Autodesk Inventor part; units mm, degrees
(part 3 of 4)
sketch "Sketch6" plane through (0, -25.4, 0) normal (0, -1, 0) x (1, 0, 0)
  line L0 (203.2, 0) -> (203.2, 304.8) projected
  line L1 (203.2, 304.8) -> (0, 304.8) projected
  line L2 (0, 304.8) -> (0, 0) projected
  line L3 (0, 0) -> (203.2, 0) projected
  line L4 (50.8, 88.9) -> (50.8, 215.9) construction
  line L5 (50.8, 215.9) -> (152.4, 215.9) construction
  line L6 (152.4, 215.9) -> (152.4, 88.9) construction
  line L7 (152.4, 88.9) -> (50.8, 88.9) construction
  spline S0 degree 2 poles (81.1955, 116.5983) (82.3959, 116.5983) (83.7001, 115.1312) (83.7001, 113.8937) knots 0 0 0 1 2 2 2
  spline S1 degree 2 poles (83.7001, 113.8937) (83.7001, 113.5973) (83.5964, 112.6117) (83.5223, 112.2783) knots 0 0 0 1 2 2 2
  line L8 (83.5223, 112.2783) -> (82.3515, 112.2783)
  line L9 (82.3515, 112.2783) -> (82.3515, 112.345)
  spline S2 degree 2 poles (82.3515, 112.345) (82.4404, 112.5969) (82.6479, 113.3453) (82.6479, 113.7307) knots 0 0 0 1 2 2 2
  spline S3 degree 2 poles (82.6479, 113.7307) (82.6479, 114.2938) (82.3885, 114.9681) (82.1514, 115.1237) knots 0 0 0 1 2 2 2
  spline S4 degree 2 poles (82.1514, 115.1237) (81.9069, 115.2942) (81.1955, 115.3831) (80.7287, 115.3831) knots 0 0 0 1 2 2 2
  line L10 (80.7287, 115.3831) -> (75.4009, 115.3831)
  line L11 (75.4009, 115.3831) -> (75.4009, 113.4491)
  line L12 (75.4009, 113.4491) -> (74.4301, 113.4491)
  line L13 (74.4301, 113.4491) -> (74.4301, 116.5983)
  line L14 (74.4301, 116.5983) -> (81.1955, 116.5983)
  spline S5 degree 2 poles (83.7668, 121.5853) (83.7668, 120.7776) (83.3444, 119.5772) (82.9221, 119.1548) knots 0 0 0 1 2 2 2
  spline S6 degree 2 poles (82.9221, 119.1548) (82.4478, 118.6732) (81.114, 118.2804) (80.1359, 118.2804) knots 0 0 0 1 2 2 2
  line L15 (80.1359, 118.2804) -> (74.4301, 118.2804)
  line L16 (74.4301, 118.2804) -> (74.4301, 119.4957)
  line L17 (74.4301, 119.4957) -> (80.1359, 119.4957)
  spline S7 degree 2 poles (80.1359, 119.4957) (80.7731, 119.4957) (81.6327, 119.6587) (81.981, 119.8884) knots 0 0 0 1 2 2 2
  spline S8 degree 2 poles (81.981, 119.8884) (82.3515, 120.1329) (82.7294, 120.9777) (82.7294, 121.5853) knots 0 0 0 1 2 2 2
  spline S9 degree 2 poles (82.7294, 121.5853) (82.7294, 122.1559) (82.3515, 123.0451) (81.981, 123.2896) knots 0 0 0 1 2 2 2
  spline S10 degree 2 poles (81.981, 123.2896) (81.6327, 123.5193) (80.7806, 123.6824) (80.1655, 123.6824) knots 0 0 0 1 2 2 2
  line L18 (80.1655, 123.6824) -> (74.4301, 123.6824)
  line L19 (74.4301, 123.6824) -> (74.4301, 124.8976)
  line L20 (74.4301, 124.8976) -> (80.1359, 124.8976)
  spline S11 degree 2 poles (80.1359, 124.8976) (81.0918, 124.8976) (82.4552, 124.5123) (82.9221, 124.0232) knots 0 0 0 1 2 2 2
  spline S12 degree 2 poles (82.9221, 124.0232) (83.3518, 123.586) (83.7668, 122.4301) (83.7668, 121.5853) knots 0 0 0 1 2 2 2
  spline S13 degree 2 poles (83.7372, 129.188) (83.7372, 128.1951) (83.3222, 126.802) (83.0258, 126.187) knots 0 0 0 1 2 2 2
  line L21 (83.0258, 126.187) -> (81.4993, 126.187)
  line L22 (81.4993, 126.187) -> (81.4993, 126.2759)
  spline S14 degree 2 poles (81.4993, 126.2759) (82.0625, 126.8761) (82.6849, 128.3951) (82.6849, 129.0991) knots 0 0 0 1 2 2 2
  spline S15 degree 2 poles (82.6849, 129.0991) (82.6849, 130.1069) (81.8476, 131.1369) (81.1585, 131.1369) knots 0 0 0 1 2 2 2
  spline S16 degree 2 poles (81.1585, 131.1369) (80.6101, 131.1369) (79.9284, 130.5959) (79.758, 130.0105) knots 0 0 0 1 2 2 2
  spline S17 degree 2 poles (79.758, 130.0105) (79.6394, 129.5882) (79.4764, 128.8842) (79.343, 128.3581) knots 0 0 0 1 2 2 2
  spline S18 degree 2 poles (79.343, 128.3581) (79.217, 127.8839) (78.8391, 127.1354) (78.5353, 126.8464) knots 0 0 0 1 2 2 2
  spline S19 degree 2 poles (78.5353, 126.8464) (78.2315, 126.5649) (77.4164, 126.2536) (76.8829, 126.2536) knots 0 0 0 1 2 2 2
  spline S20 degree 2 poles (76.8829, 126.2536) (75.7714, 126.2536) (74.2671, 127.9876) (74.2671, 129.3288) knots 0 0 0 1 2 2 2
  spline S21 degree 2 poles (74.2671, 129.3288) (74.2671, 130.0995) (74.5709, 131.4629) (74.8599, 132.0483) knots 0 0 0 1 2 2 2
  line L23 (74.8599, 132.0483) -> (76.3123, 132.0483)
  line L24 (76.3123, 132.0483) -> (76.3123, 131.9594)
  spline S22 degree 2 poles (76.3123, 131.9594) (75.9122, 131.5222) (75.3194, 130.1587) (75.3194, 129.4103) knots 0 0 0 1 2 2 2
  spline S23 degree 2 poles (75.3194, 129.4103) (75.3194, 128.5656) (76.1122, 127.5208) (76.7569, 127.5208) knots 0 0 0 1 2 2 2
  spline S24 degree 2 poles (76.7569, 127.5208) (77.3349, 127.5208) (78.024, 128.1358) (78.1796, 128.7138) knots 0 0 0 1 2 2 2
  spline S25 degree 2 poles (78.1796, 128.7138) (78.2834, 129.0991) (78.5501, 130.218) (78.6613, 130.5885) knots 0 0 0 1 2 2 2
  spline S26 degree 2 poles (78.6613, 130.5885) (78.9503, 131.5296) (80.1137, 132.404) (80.9658, 132.404) knots 0 0 0 1 2 2 2
  spline S27 degree 2 poles (80.9658, 132.404) (81.5067, 132.404) (82.5441, 131.9668) (82.9072, 131.5741) knots 0 0 0 1 2 2 2
  spline S28 degree 2 poles (82.9072, 131.5741) (83.3074, 131.1369) (83.7372, 130.0254) (83.7372, 129.188) knots 0 0 0 1 2 2 2
  line L25 (83.5741, 135.7756) -> (75.512, 135.7756)
  line L26 (75.512, 135.7756) -> (75.512, 132.7078)
  line L27 (75.512, 132.7078) -> (74.4301, 132.7078)
  line L28 (74.4301, 132.7078) -> (74.4301, 140.0586)
  line L29 (74.4301, 140.0586) -> (75.512, 140.0586)
  line L30 (75.512, 140.0586) -> (75.512, 136.9908)
  line L31 (75.512, 136.9908) -> (83.5741, 136.9908)
  line L32 (83.5741, 136.9908) -> (83.5741, 135.7756)
  line L33 (83.5741, 144.1711) -> (83.5741, 140.6291)
  line L34 (83.5741, 140.6291) -> (82.6405, 140.6291)
  line L35 (82.6405, 140.6291) -> (82.6405, 141.7925)
  line L36 (82.6405, 141.7925) -> (75.3638, 141.7925)
  line L37 (75.3638, 141.7925) -> (75.3638, 140.6291)
  line L38 (75.3638, 140.6291) -> (74.4301, 140.6291)
  line L39 (74.4301, 140.6291) -> (74.4301, 144.1711)
  line L40 (74.4301, 144.1711) -> (75.3638, 144.1711)
  line L41 (75.3638, 144.1711) -> (75.3638, 143.0078)
  line L42 (75.3638, 143.0078) -> (82.6405, 143.0078)
  line L43 (82.6405, 143.0078) -> (82.6405, 144.1711)
  line L44 (82.6405, 144.1711) -> (83.5741, 144.1711)
  line L45 (83.5741, 152.2185) -> (83.5741, 150.855)
  line L46 (83.5741, 150.855) -> (75.6899, 146.8091)
  line L47 (75.6899, 146.8091) -> (83.5741, 146.8091)
  line L48 (83.5741, 146.8091) -> (83.5741, 145.6754)
  line L49 (83.5741, 145.6754) -> (74.4301, 145.6754)
  line L50 (74.4301, 145.6754) -> (74.4301, 147.4019)
  line L51 (74.4301, 147.4019) -> (81.6698, 151.0847)
  line L52 (81.6698, 151.0847) -> (74.4301, 151.0847)
  line L53 (74.4301, 151.0847) -> (74.4301, 152.2185)
  line L54 (74.4301, 152.2185) -> (83.5741, 152.2185)
  line L55 (83.5741, 157.0128) -> (74.4301, 160.0953)
  line L56 (74.4301, 160.0953) -> (74.4301, 161.5922)
  line L57 (74.4301, 161.5922) -> (83.5741, 164.6747)
  line L58 (83.5741, 164.6747) -> (83.5741, 163.3928)
  line L59 (83.5741, 163.3928) -> (81.0177, 162.5629)
  line L60 (81.0177, 162.5629) -> (81.0177, 159.0727)
  line L61 (81.0177, 159.0727) -> (83.5741, 158.2428)
  line L62 (83.5741, 158.2428) -> (83.5741, 157.0128)
  line L63 (79.9803, 162.2294) -> (75.675, 160.8141)
  line L64 (75.675, 160.8141) -> (79.9803, 159.4062)
  line L65 (79.9803, 159.4062) -> (79.9803, 162.2294)
  line L66 (83.5741, 170.8399) -> (83.5741, 165.5417)
  line L67 (83.5741, 165.5417) -> (74.4301, 165.5417)
  line L68 (74.4301, 165.5417) -> (74.4301, 166.757)
  line L69 (74.4301, 166.757) -> (82.4923, 166.757)
  line L70 (82.4923, 166.757) -> (82.4923, 170.8399)
  line L71 (82.4923, 170.8399) -> (83.5741, 170.8399)
  line L72 (83.5741, 177.094) -> (83.5741, 171.7958)
  line L73 (83.5741, 171.7958) -> (74.4301, 171.7958)
  line L74 (74.4301, 171.7958) -> (74.4301, 173.011)
  line L75 (74.4301, 173.011) -> (82.4923, 173.011)
  line L76 (82.4923, 173.011) -> (82.4923, 177.094)
  line L77 (82.4923, 177.094) -> (83.5741, 177.094)
  line L78 (83.5741, 178.0499) -> (74.4301, 178.0499)
  line L79 (74.4301, 178.0499) -> (74.4301, 183.7704)
  line L80 (74.4301, 183.7704) -> (75.512, 183.7704)
  line L81 (75.512, 183.7704) -> (75.512, 179.2651)
  line L82 (75.512, 179.2651) -> (78.0166, 179.2651)
  line L83 (78.0166, 179.2651) -> (78.0166, 183.4666)
  line L84 (78.0166, 183.4666) -> (79.0985, 183.4666)
  line L85 (79.0985, 183.4666) -> (79.0985, 179.2651)
  line L86 (79.0985, 179.2651) -> (82.4923, 179.2651)
  line L87 (82.4923, 179.2651) -> (82.4923, 183.7704)
  line L88 (82.4923, 183.7704) -> (83.5741, 183.7704)
  line L89 (83.5741, 183.7704) -> (83.5741, 178.0499)
  line L90 (83.5741, 191.6473) -> (83.5741, 190.2839)
  line L91 (83.5741, 190.2839) -> (75.6899, 186.238)
  line L92 (75.6899, 186.238) -> (83.5741, 186.238)
  line L93 (83.5741, 186.238) -> (83.5741, 185.1042)
  line L94 (83.5741, 185.1042) -> (74.4301, 185.1042)
  line L95 (74.4301, 185.1042) -> (74.4301, 186.8308)
  line L96 (74.4301, 186.8308) -> (81.6698, 190.5136)
  line L97 (81.6698, 190.5136) -> (74.4301, 190.5136)
  line L98 (74.4301, 190.5136) -> (74.4301, 191.6473)
  line L99 (74.4301, 191.6473) -> (83.5741, 191.6473)
  line L100 (98.6295, 121.1222) -> (89.4855, 124.2048)
  line L101 (89.4855, 124.2048) -> (89.4855, 125.7016)
  line L102 (89.4855, 125.7016) -> (98.6295, 128.7842)
  line L103 (98.6295, 128.7842) -> (98.6295, 127.5022)
  line L104 (98.6295, 127.5022) -> (96.073, 126.6723)
  line L105 (96.073, 126.6723) -> (96.073, 123.1822)
  line L106 (96.073, 123.1822) -> (98.6295, 122.3523)
  line L107 (98.6295, 122.3523) -> (98.6295, 121.1222)
  line L108 (95.0356, 126.3389) -> (90.7304, 124.9235)
  line L109 (90.7304, 124.9235) -> (95.0356, 123.5156)
  line L110 (95.0356, 123.5156) -> (95.0356, 126.3389)
  line L111 (98.6295, 134.5714) -> (98.6295, 130.1106)
  line L112 (98.6295, 130.1106) -> (97.6958, 130.1106)
  line L113 (97.6958, 130.1106) -> (97.6958, 131.7704)
  line L114 (97.6958, 131.7704) -> (91.5677, 131.7704)
  line L115 (91.5677, 131.7704) -> (91.5677, 130.1106)
  line L116 (91.5677, 130.1106) -> (90.7304, 130.1106)
  spline S29 degree 2 poles (90.7304, 130.1106) (90.7304, 131.0516) (90.1969, 131.9409) (89.4559, 132.0001) knots 0 0 0 1 2 2 2
  line L117 (89.4559, 132.0001) -> (89.4559, 132.9486)
  line L118 (89.4559, 132.9486) -> (97.6958, 132.9486)
  line L119 (97.6958, 132.9486) -> (97.6958, 134.5714)
  line L120 (97.6958, 134.5714) -> (98.6295, 134.5714)
  line L121 (95.4876, 142.1371) -> (95.4876, 141.0478)
  line L122 (95.4876, 141.0478) -> (98.6295, 141.0478)
  line L123 (98.6295, 141.0478) -> (98.6295, 139.8696)
  line L124 (98.6295, 139.8696) -> (95.4876, 139.8696)
  line L125 (95.4876, 139.8696) -> (95.4876, 135.8311)
  line L126 (95.4876, 135.8311) -> (94.1983, 135.8311)
  line L127 (94.1983, 135.8311) -> (89.4855, 139.9215)
  line L128 (89.4855, 139.9215) -> (89.4855, 141.0478)
  line L129 (89.4855, 141.0478) -> (94.5021, 141.0478)
  line L130 (94.5021, 141.0478) -> (94.5021, 142.1371)
  line L131 (94.5021, 142.1371) -> (95.4876, 142.1371)
  line L132 (94.5021, 139.8696) -> (90.9305, 139.8696)
  line L133 (90.9305, 139.8696) -> (94.5021, 136.7944)
  line L134 (94.5021, 136.7944) -> (94.5021, 139.8696)
  spline S30 degree 2 poles (95.7248, 148.6579) (96.3843, 148.6579) (97.5106, 148.2356) (97.9255, 147.8502) knots 0 0 0 1 2 2 2
  spline S31 degree 2 poles (97.9255, 147.8502) (98.3405, 147.4649) (98.8222, 146.3163) (98.8222, 145.605) knots 0 0 0 1 2 2 2
  spline S32 degree 2 poles (98.8222, 145.605) (98.8222, 144.9529) (98.5332, 143.6784) (98.3035, 143.2115) knots 0 0 0 1 2 2 2
  line L135 (98.3035, 143.2115) -> (97.0067, 143.2115)
  line L136 (97.0067, 143.2115) -> (97.0067, 143.3005)
  spline S33 degree 2 poles (97.0067, 143.3005) (97.1104, 143.4412) (97.3772, 143.9674) (97.4958, 144.286) knots 0 0 0 1 2 2 2
  spline S34 degree 2 poles (97.4958, 144.286) (97.6217, 144.6491) (97.7625, 145.2493) (97.7625, 145.6272) knots 0 0 0 1 2 2 2
  spline S35 degree 2 poles (97.7625, 145.6272) (97.7625, 145.9977) (97.4958, 146.6943) (97.2068, 146.9462) knots 0 0 0 1 2 2 2
  spline S36 degree 2 poles (97.2068, 146.9462) (96.9326, 147.1759) (96.2064, 147.413) (95.7174, 147.413) knots 0 0 0 1 2 2 2
  spline S37 degree 2 poles (95.7174, 147.413) (95.2283, 147.413) (94.6058, 147.1463) (94.3984, 146.8943) knots 0 0 0 1 2 2 2
  spline S38 degree 2 poles (94.3984, 146.8943) (94.1687, 146.635) (93.976, 145.8643) (93.976, 145.3975) knots 0 0 0 1 2 2 2
  spline S39 degree 2 poles (93.976, 145.3975) (93.976, 144.8936) (94.1316, 143.8933) (94.1983, 143.5895) knots 0 0 0 1 2 2 2
  line L137 (94.1983, 143.5895) -> (89.4855, 143.5895)
  line L138 (89.4855, 143.5895) -> (89.4855, 148.6061)
  line L139 (89.4855, 148.6061) -> (90.56, 148.6061)
  line L140 (90.56, 148.6061) -> (90.56, 144.7676)
  line L141 (90.56, 144.7676) -> (92.9979, 144.7676)
  spline S40 degree 2 poles (92.9979, 144.7676) (92.9682, 144.9899) (92.946, 145.4197) (92.946, 145.5976) knots 0 0 0 1 2 2 2
  spline S41 degree 2 poles (92.946, 145.5976) (92.946, 146.3015) (93.1757, 147.2722) (93.5166, 147.7168) knots 0 0 0 1 2 2 2
  spline S42 degree 2 poles (93.5166, 147.7168) (93.8574, 148.1689) (94.8948, 148.6579) (95.7248, 148.6579) knots 0 0 0 1 2 2 2
  spline S43 degree 2 poles (95.6655, 155.7568) (96.3694, 155.7568) (97.5625, 155.2899) (97.9626, 154.8972) knots 0 0 0 1 2 2 2
  spline S44 degree 2 poles (97.9626, 154.8972) (98.385, 154.4896) (98.8222, 153.467) (98.8222, 152.852) knots 0 0 0 1 2 2 2
  spline S45 degree 2 poles (98.8222, 152.852) (98.8222, 152.237) (98.4072, 151.2218) (97.9922, 150.8365) knots 0 0 0 1 2 2 2
  spline S46 degree 2 poles (97.9922, 150.8365) (97.4958, 150.3622) (95.8285, 149.8287) (94.6133, 149.8287) knots 0 0 0 1 2 2 2
  spline S47 degree 2 poles (94.6133, 149.8287) (93.4202, 149.8287) (91.501, 150.3178) (90.7897, 150.8291) knots 0 0 0 1 2 2 2
  spline S48 degree 2 poles (90.7897, 150.8291) (90.0931, 151.3255) (89.3151, 152.8965) (89.3151, 153.9265) knots 0 0 0 1 2 2 2
  spline S49 degree 2 poles (89.3151, 153.9265) (89.3151, 154.2303) (89.3744, 154.7638) (89.441, 154.9639) knots 0 0 0 1 2 2 2
  line L142 (89.441, 154.9639) -> (90.6192, 154.9639)
  line L143 (90.6192, 154.9639) -> (90.6192, 154.912)
  spline S50 degree 2 poles (90.6192, 154.912) (90.5303, 154.7416) (90.3747, 154.1191) (90.3747, 153.7634) knots 0 0 0 1 2 2 2
  spline S51 degree 2 poles (90.3747, 153.7634) (90.3747, 152.6223) (91.916, 151.2218) (93.4276, 151.0884) knots 0 0 0 1 2 2 2
  spline S52 degree 2 poles (93.4276, 151.0884) (93.1238, 151.5256) (92.7904, 152.4445) (92.7904, 152.9928) knots 0 0 0 1 2 2 2
  spline S53 degree 2 poles (92.7904, 152.9928) (92.7904, 153.5263) (93.0053, 154.3266) (93.3313, 154.7638) knots 0 0 0 1 2 2 2
  spline S54 degree 2 poles (93.3313, 154.7638) (93.7092, 155.2677) (94.88, 155.7568) (95.6655, 155.7568) knots 0 0 0 1 2 2 2
  spline S55 degree 2 poles (95.7174, 154.5119) (95.1542, 154.5119) (94.391, 154.2155) (94.1242, 153.8894) knots 0 0 0 1 2 2 2
  spline S56 degree 2 poles (94.1242, 153.8894) (93.9315, 153.6449) (93.8056, 153.0373) (93.8056, 152.7186) knots 0 0 0 1 2 2 2
  spline S57 degree 2 poles (93.8056, 152.7186) (93.8056, 152.2888) (94.0649, 151.4812) (94.3094, 151.0884) knots 0 0 0 1 2 2 2
  spline S58 degree 2 poles (94.3094, 151.0884) (94.4428, 151.081) (94.6948, 151.0662) (94.8874, 151.0662) knots 0 0 0 1 2 2 2
  spline S59 degree 2 poles (94.8874, 151.0662) (95.8359, 151.0662) (96.9993, 151.4367) (97.3031, 151.7183) knots 0 0 0 1 2 2 2
  spline S60 degree 2 poles (97.3031, 151.7183) (97.5921, 151.9776) (97.8218, 152.5408) (97.8218, 152.8594) knots 0 0 0 1 2 2 2
  spline S61 degree 2 poles (97.8218, 152.8594) (97.8218, 153.6004) (96.7696, 154.5119) (95.7174, 154.5119) knots 0 0 0 1 2 2 2
  spline S62 degree 2 poles (95.6655, 162.6185) (96.3694, 162.6185) (97.5625, 162.1516) (97.9626, 161.7589) knots 0 0 0 1 2 2 2
  spline S63 degree 2 poles (97.9626, 161.7589) (98.385, 161.3513) (98.8222, 160.3288) (98.8222, 159.7137) knots 0 0 0 1 2 2 2
  spline S64 degree 2 poles (98.8222, 159.7137) (98.8222, 159.0987) (98.4072, 158.0835) (97.9922, 157.6982) knots 0 0 0 1 2 2 2
  spline S65 degree 2 poles (97.9922, 157.6982) (97.4958, 157.2239) (95.8285, 156.6904) (94.6133, 156.6904) knots 0 0 0 1 2 2 2
  spline S66 degree 2 poles (94.6133, 156.6904) (93.4202, 156.6904) (91.501, 157.1795) (90.7897, 157.6908) knots 0 0 0 1 2 2 2
  spline S67 degree 2 poles (90.7897, 157.6908) (90.0931, 158.1872) (89.3151, 159.7582) (89.3151, 160.7882) knots 0 0 0 1 2 2 2
  spline S68 degree 2 poles (89.3151, 160.7882) (89.3151, 161.092) (89.3744, 161.6255) (89.441, 161.8256) knots 0 0 0 1 2 2 2
  line L144 (89.441, 161.8256) -> (90.6192, 161.8256)
  line L145 (90.6192, 161.8256) -> (90.6192, 161.7737)
  spline S69 degree 2 poles (90.6192, 161.7737) (90.5303, 161.6033) (90.3747, 160.9808) (90.3747, 160.6252) knots 0 0 0 1 2 2 2
  spline S70 degree 2 poles (90.3747, 160.6252) (90.3747, 159.484) (91.916, 158.0835) (93.4276, 157.9501) knots 0 0 0 1 2 2 2
  spline S71 degree 2 poles (93.4276, 157.9501) (93.1238, 158.3873) (92.7904, 159.3062) (92.7904, 159.8545) knots 0 0 0 1 2 2 2
  spline S72 degree 2 poles (92.7904, 159.8545) (92.7904, 160.388) (93.0053, 161.1883) (93.3313, 161.6255) knots 0 0 0 1 2 2 2
  spline S73 degree 2 poles (93.3313, 161.6255) (93.7092, 162.1294) (94.88, 162.6185) (95.6655, 162.6185) knots 0 0 0 1 2 2 2
  spline S74 degree 2 poles (95.7174, 161.3736) (95.1542, 161.3736) (94.391, 161.0772) (94.1242, 160.7511) knots 0 0 0 1 2 2 2
  spline S75 degree 2 poles (94.1242, 160.7511) (93.9315, 160.5066) (93.8056, 159.899) (93.8056, 159.5803) knots 0 0 0 1 2 2 2
  spline S76 degree 2 poles (93.8056, 159.5803) (93.8056, 159.1506) (94.0649, 158.3429) (94.3094, 157.9501) knots 0 0 0 1 2 2 2
  spline S77 degree 2 poles (94.3094, 157.9501) (94.4428, 157.9427) (94.6948, 157.9279) (94.8874, 157.9279) knots 0 0 0 1 2 2 2
  spline S78 degree 2 poles (94.8874, 157.9279) (95.8359, 157.9279) (96.9993, 158.2984) (97.3031, 158.58) knots 0 0 0 1 2 2 2
  spline S79 degree 2 poles (97.3031, 158.58) (97.5921, 158.8393) (97.8218, 159.4025) (97.8218, 159.7211) knots 0 0 0 1 2 2 2
  spline S80 degree 2 poles (97.8218, 159.7211) (97.8218, 160.4621) (96.7696, 161.3736) (95.7174, 161.3736) knots 0 0 0 1 2 2 2
  spline S81 degree 2 poles (94.0575, 169.3912) (96.5176, 169.3912) (98.8222, 167.9611) (98.8222, 166.4717) knots 0 0 0 1 2 2 2
  spline S82 degree 2 poles (98.8222, 166.4717) (98.8222, 164.96) (96.4732, 163.5447) (94.0649, 163.5447) knots 0 0 0 1 2 2 2
  spline S83 degree 2 poles (94.0649, 163.5447) (91.59, 163.5447) (89.3002, 164.9749) (89.3002, 166.4717) knots 0 0 0 1 2 2 2
  spline S84 degree 2 poles (89.3002, 166.4717) (89.3002, 167.9759) (91.6715, 169.3912) (94.0575, 169.3912) knots 0 0 0 1 2 2 2
  spline S85 degree 2 poles (96.8437, 167.8203) (96.3917, 167.9982) (94.9986, 168.1464) (94.0575, 168.1464) knots 0 0 0 1 2 2 2
  spline S86 degree 2 poles (94.0575, 168.1464) (93.1164, 168.1464) (91.7307, 167.9982) (91.2639, 167.8129) knots 0 0 0 1 2 2 2
  spline S87 degree 2 poles (91.2639, 167.8129) (90.7971, 167.6276) (90.3154, 166.983) (90.3154, 166.4717) knots 0 0 0 1 2 2 2
  spline S88 degree 2 poles (90.3154, 166.4717) (90.3154, 165.9604) (90.7971, 165.3009) (91.2787, 165.1082) knots 0 0 0 1 2 2 2
  spline S89 degree 2 poles (91.2787, 165.1082) (91.7456, 164.923) (93.1683, 164.7896) (94.0649, 164.7896) knots 0 0 0 1 2 2 2
  spline S90 degree 2 poles (94.0649, 164.7896) (95.0282, 164.7896) (96.3176, 164.9082) (96.8214, 165.1008) knots 0 0 0 1 2 2 2
  spline S91 degree 2 poles (96.8214, 165.1008) (97.2957, 165.2787) (97.807, 165.9382) (97.807, 166.4717) knots 0 0 0 1 2 2 2
  spline S92 degree 2 poles (97.807, 166.4717) (97.807, 166.9756) (97.3253, 167.6351) (96.8437, 167.8203) knots 0 0 0 1 2 2 2
  line L146 (90.8564, 176.3048) -> (98.6295, 172.3478)
  line L147 (98.6295, 172.3478) -> (98.6295, 171.0437)
  line L148 (98.6295, 171.0437) -> (90.56, 175.2229)
  line L149 (90.56, 175.2229) -> (90.56, 170.5027)
  line L150 (90.56, 170.5027) -> (89.4855, 170.5027)
  line L151 (89.4855, 170.5027) -> (89.4855, 176.3048)
  line L152 (89.4855, 176.3048) -> (90.8564, 176.3048)
  line L153 (98.6295, 182.6034) -> (98.6295, 178.1425)
  line L154 (98.6295, 178.1425) -> (97.6958, 178.1425)
  line L155 (97.6958, 178.1425) -> (97.6958, 179.8024)
  line L156 (97.6958, 179.8024) -> (91.5677, 179.8024)
  line L157 (91.5677, 179.8024) -> (91.5677, 178.1425)
  line L158 (91.5677, 178.1425) -> (90.7304, 178.1425)
  spline S93 degree 2 poles (90.7304, 178.1425) (90.7304, 179.0836) (90.1969, 179.9728) (89.4559, 180.0321) knots 0 0 0 1 2 2 2
  line L159 (89.4559, 180.0321) -> (89.4559, 180.9806)
  line L160 (89.4559, 180.9806) -> (97.6958, 180.9806)
  line L161 (97.6958, 180.9806) -> (97.6958, 182.6034)
  line L162 (97.6958, 182.6034) -> (98.6295, 182.6034)
  spline S94 degree 2 poles (113.8775, 106.2724) (115.0483, 106.2724) (116.2784, 105.0127) (116.2784, 103.9086) knots 0 0 0 1 2 2 2
  spline S95 degree 2 poles (116.2784, 103.9086) (116.2784, 103.716) (116.2413, 103.2417) (116.2043, 103.012) knots 0 0 0 1 2 2 2
  line L163 (116.2043, 103.012) -> (115.1669, 103.012)
  line L164 (115.1669, 103.012) -> (115.1669, 103.0787)
  spline S96 degree 2 poles (115.1669, 103.0787) (115.1965, 103.2121) (115.2558, 103.5381) (115.2558, 103.6863) knots 0 0 0 1 2 2 2
  spline S97 degree 2 poles (115.2558, 103.6863) (115.2558, 104.1458) (115.0261, 104.746) (114.7815, 104.8868) knots 0 0 0 1 2 2 2
  spline S98 degree 2 poles (114.7815, 104.8868) (114.5592, 105.0276) (113.8849, 105.1165) (113.4033, 105.1165) knots 0 0 0 1 2 2 2
  line L165 (113.4033, 105.1165) -> (107.779, 105.1165)
  line L166 (107.779, 105.1165) -> (107.779, 103.879)
  line L167 (107.779, 103.879) -> (106.8232, 103.879)
  line L168 (106.8232, 103.879) -> (106.8232, 106.2724)
  line L169 (106.8232, 106.2724) -> (113.8775, 106.2724)
  line L170 (105.682, 106.2799) -> (105.682, 104.9683)
  line L171 (105.682, 104.9683) -> (104.4816, 104.9683)
  line L172 (104.4816, 104.9683) -> (104.4816, 106.2799)
  line L173 (104.4816, 106.2799) -> (105.682, 106.2799)
  spline S99 degree 2 poles (110.1429, 113.6973) (111.8249, 113.6973) (113.8775, 112.0671) (113.8775, 110.837) knots 0 0 0 1 2 2 2
  spline S100 degree 2 poles (113.8775, 110.837) (113.8775, 110.2813) (113.6033, 109.4884) (113.3662, 109.1031) knots 0 0 0 1 2 2 2
  line L174 (113.3662, 109.1031) -> (113.6849, 109.029)
  line L175 (113.6849, 109.029) -> (113.6849, 107.9471)
  line L176 (113.6849, 107.9471) -> (104.1333, 107.9471)
  line L177 (104.1333, 107.9471) -> (104.1333, 109.1031)
  line L178 (104.1333, 109.1031) -> (107.5419, 109.1031)
  spline S101 degree 2 poles (107.5419, 109.1031) (107.1492, 109.5403) (106.6305, 110.5555) (106.6305, 111.2001) knots 0 0 0 1 2 2 2
  spline S102 degree 2 poles (106.6305, 111.2001) (106.6305, 112.3635) (108.4904, 113.6973) (110.1429, 113.6973) knots 0 0 0 1 2 2 2
  spline S103 degree 2 poles (110.2318, 112.5043) (109.0017, 112.5043) (107.7272, 111.7559) (107.7272, 110.926) knots 0 0 0 1 2 2 2
  spline S104 degree 2 poles (107.7272, 110.926) (107.7272, 110.4591) (108.1718, 109.4958) (108.5126, 109.1031) knots 0 0 0 1 2 2 2
  line L179 (108.5126, 109.1031) -> (112.4474, 109.1031)
  spline S105 degree 2 poles (112.4474, 109.1031) (112.6623, 109.5403) (112.8401, 110.2146) (112.8401, 110.6147) knots 0 0 0 1 2 2 2
  spline S106 degree 2 poles (112.8401, 110.6147) (112.8401, 111.4965) (111.5878, 112.5043) (110.2318, 112.5043) knots 0 0 0 1 2 2 2
  spline S107 degree 2 poles (112.9587, 118.7213) (113.0624, 118.5805) (113.4329, 118.1063) (113.5441, 117.884) knots 0 0 0 1 2 2 2
  spline S108 degree 2 poles (113.5441, 117.884) (113.7071, 117.5802) (113.8775, 117.0096) (113.8775, 116.4909) knots 0 0 0 1 2 2 2
  spline S109 degree 2 poles (113.8775, 116.4909) (113.8775, 116.0685) (113.5589, 115.3053) (113.2699, 115.0163) knots 0 0 0 1 2 2 2
  spline S110 degree 2 poles (113.2699, 115.0163) (112.9883, 114.7421) (112.1584, 114.4087) (111.699, 114.4087) knots 0 0 0 1 2 2 2
  spline S111 degree 2 poles (111.699, 114.4087) (110.9876, 114.4087) (109.9798, 115.0089) (109.6908, 115.661) knots 0 0 0 1 2 2 2
  spline S112 degree 2 poles (109.6908, 115.661) (109.4241, 116.239) (109.224, 117.8099) (109.1721, 118.7213) knots 0 0 0 1 2 2 2
  line L180 (109.1721, 118.7213) -> (108.9498, 118.7213)
  spline S113 degree 2 poles (108.9498, 118.7213) (108.5497, 118.7213) (108.0532, 118.4768) (107.9124, 118.2545) knots 0 0 0 1 2 2 2
  spline S114 degree 2 poles (107.9124, 118.2545) (107.7716, 118.0322) (107.6827, 117.3949) (107.6827, 117.0541) knots 0 0 0 1 2 2 2
  spline S115 degree 2 poles (107.6827, 117.0541) (107.6827, 116.6539) (107.9198, 115.5721) (108.1495, 115.0311) knots 0 0 0 1 2 2 2
  line L181 (108.1495, 115.0311) -> (108.1495, 114.9644)
  line L182 (108.1495, 114.9644) -> (106.9714, 114.9644)
  spline S116 degree 2 poles (106.9714, 114.9644) (106.8824, 115.2831) (106.6601, 116.4761) (106.6601, 117.0615) knots 0 0 0 1 2 2 2
  spline S117 degree 2 poles (106.6601, 117.0615) (106.6601, 117.7728) (106.8824, 118.7436) (107.1714, 119.1289) knots 0 0 0 1 2 2 2
  spline S118 degree 2 poles (107.1714, 119.1289) (107.453, 119.5068) (108.3496, 119.8773) (108.9943, 119.8773) knots 0 0 0 1 2 2 2
  line L183 (108.9943, 119.8773) -> (113.6849, 119.8773)
  line L184 (113.6849, 119.8773) -> (113.6849, 118.7213)
  line L185 (113.6849, 118.7213) -> (112.9587, 118.7213)
  line L186 (111.9954, 118.7213) -> (110.091, 118.7213)
  spline S119 degree 2 poles (110.091, 118.7213) (110.128, 118.3064) (110.254, 117.0541) (110.3726, 116.6613) knots 0 0 0 1 2 2 2
  spline S120 degree 2 poles (110.3726, 116.6613) (110.5134, 116.2019) (111.0987, 115.6017) (111.6175, 115.6017) knots 0 0 0 1 2 2 2
  spline S121 degree 2 poles (111.6175, 115.6017) (112.2103, 115.6017) (112.8105, 116.2686) (112.8105, 116.9059) knots 0 0 0 1 2 2 2
  spline S122 degree 2 poles (112.8105, 116.9059) (112.8105, 117.4468) (112.3436, 118.336) (111.9954, 118.7213) knots 0 0 0 1 2 2 2
  line L187 (113.6849, 122.6783) -> (113.6849, 121.5223)
  line L188 (113.6849, 121.5223) -> (104.1333, 121.5223)
  line L189 (104.1333, 121.5223) -> (104.1333, 122.6783)
  line L190 (104.1333, 122.6783) -> (113.6849, 122.6783)
  line L191 (113.6849, 125.5534) -> (113.6849, 124.3974)
  line L192 (113.6849, 124.3974) -> (104.1333, 124.3974)
  line L193 (104.1333, 124.3974) -> (104.1333, 125.5534)
  line L194 (104.1333, 125.5534) -> (113.6849, 125.5534)
  spline S123 degree 2 poles (113.8405, 130.2291) (113.8405, 128.5841) (111.9954, 126.7761) (110.2911, 126.7761) knots 0 0 0 1 2 2 2
  spline S124 degree 2 poles (110.2911, 126.7761) (108.6164, 126.7761) (106.6305, 128.5322) (106.6305, 129.9476) knots 0 0 0 1 2 2 2
  spline S125 degree 2 poles (106.6305, 129.9476) (106.6305, 130.5848) (107.001, 131.5704) (107.3937, 131.9334) knots 0 0 0 1 2 2 2
  spline S126 degree 2 poles (107.3937, 131.9334) (107.7865, 132.3039) (108.9202, 132.6967) (109.7427, 132.6967) knots 0 0 0 1 2 2 2
  line L195 (109.7427, 132.6967) -> (110.3726, 132.6967)
  line L196 (110.3726, 132.6967) -> (110.3726, 127.9468)
  spline S127 degree 2 poles (110.3726, 127.9468) (111.5656, 127.9468) (112.8327, 129.1473) (112.8327, 130.2143) knots 0 0 0 1 2 2 2
  spline S128 degree 2 poles (112.8327, 130.2143) (112.8327, 130.5922) (112.6623, 131.3258) (112.5289, 131.6222) knots 0 0 0 1 2 2 2
  spline S129 degree 2 poles (112.5289, 131.6222) (112.3807, 131.9334) (112.1213, 132.3632) (112.0028, 132.504) knots 0 0 0 1 2 2 2
  line L197 (112.0028, 132.504) -> (112.0028, 132.5707)
  line L198 (112.0028, 132.5707) -> (113.2625, 132.5707)
  spline S130 degree 2 poles (113.2625, 132.5707) (113.344, 132.3706) (113.5811, 131.763) (113.6478, 131.5259) knots 0 0 0 1 2 2 2
  spline S131 degree 2 poles (113.6478, 131.5259) (113.7441, 131.1924) (113.8405, 130.6441) (113.8405, 130.2291) knots 0 0 0 1 2 2 2
  spline S132 degree 2 poles (109.4908, 131.5704) (109.0239, 131.5555) (108.3422, 131.3629) (108.1125, 131.1776) knots 0 0 0 1 2 2 2
  spline S133 degree 2 poles (108.1125, 131.1776) (107.8531, 130.9776) (107.579, 130.3477) (107.579, 129.8809) knots 0 0 0 1 2 2 2
  spline S134 degree 2 poles (107.579, 129.8809) (107.579, 129.4214) (107.8531, 128.7768) (108.1199, 128.51) knots 0 0 0 1 2 2 2
  spline S135 degree 2 poles (108.1199, 128.51) (108.3941, 128.2507) (109.0536, 127.9839) (109.4908, 127.9468) knots 0 0 0 1 2 2 2
  line L199 (109.4908, 127.9468) -> (109.4908, 131.5704)
  line L200 (113.6849, 139.2546) -> (113.6849, 138.0986)
  line L201 (113.6849, 138.0986) -> (109.7724, 138.0986)
  spline S136 degree 2 poles (109.7724, 138.0986) (109.2981, 138.0986) (108.483, 138.0097) (108.2385, 137.8763) knots 0 0 0 1 2 2 2
  spline S137 degree 2 poles (108.2385, 137.8763) (107.9791, 137.7355) (107.7272, 137.2316) (107.7272, 136.8018) knots 0 0 0 1 2 2 2
  spline S138 degree 2 poles (107.7272, 136.8018) (107.7272, 136.3721) (108.1866, 135.4606) (108.5571, 135.0234) knots 0 0 0 1 2 2 2
  line L202 (108.5571, 135.0234) -> (113.6849, 135.0234)
  line L203 (113.6849, 135.0234) -> (113.6849, 133.8675)
  line L204 (113.6849, 133.8675) -> (106.8232, 133.8675)
  line L205 (106.8232, 133.8675) -> (106.8232, 135.0234)
  line L206 (106.8232, 135.0234) -> (107.5864, 135.0234)
  spline S139 degree 2 poles (107.5864, 135.0234) (107.1196, 135.5421) (106.6305, 136.5425) (106.6305, 137.1057) knots 0 0 0 1 2 2 2
  spline S140 degree 2 poles (106.6305, 137.1057) (106.6305, 138.1134) (107.9643, 139.2546) (109.2314, 139.2546) knots 0 0 0 1 2 2 2
  line L207 (109.2314, 139.2546) -> (113.6849, 139.2546)
  spline S141 degree 2 poles (109.6093, 150.7179) (110.4615, 150.7179) (112.0546, 150.2511) (112.7141, 149.8139) knots 0 0 0 1 2 2 2
  line L208 (112.7141, 149.8139) -> (112.7141, 147.2352)
  line L209 (112.7141, 147.2352) -> (112.0028, 147.0796)
  spline S142 degree 2 poles (112.0028, 147.0796) (112.351, 146.6646) (112.766, 145.9755) (112.766, 145.3753) knots 0 0 0 1 2 2 2
  spline S143 degree 2 poles (112.766, 145.3753) (112.766, 144.4342) (111.2469, 143.2264) (109.8094, 143.2264) knots 0 0 0 1 2 2 2
  spline S144 degree 2 poles (109.8094, 143.2264) (108.3644, 143.2264) (106.7565, 144.7084) (106.7565, 145.6643) knots 0 0 0 1 2 2 2
  spline S145 degree 2 poles (106.7565, 145.6643) (106.7565, 146.1089) (106.9788, 146.7461) (107.164, 147.0722) knots 0 0 0 1 2 2 2
  line L210 (107.164, 147.0722) -> (106.8676, 147.0722)
  line L211 (106.8676, 147.0722) -> (106.8676, 148.0429)
  line L212 (106.8676, 148.0429) -> (112.0324, 148.0429)
  line L213 (112.0324, 148.0429) -> (112.0324, 149.436)
  spline S146 degree 2 poles (112.0324, 149.436) (111.5952, 149.6731) (110.2095, 149.8732) (109.6464, 149.8732) knots 0 0 0 1 2 2 2
  spline S147 degree 2 poles (109.6464, 149.8732) (107.6383, 149.8732) (105.1929, 147.828) (105.1929, 145.9088) knots 0 0 0 1 2 2 2
  spline S148 degree 2 poles (105.1929, 145.9088) (105.1929, 144.0933) (107.8383, 141.7295) (109.7279, 141.7295) knots 0 0 0 1 2 2 2
  spline S149 degree 2 poles (109.7279, 141.7295) (111.7508, 141.7295) (114.2628, 144.0266) (114.2628, 145.8792) knots 0 0 0 1 2 2 2
  spline S150 degree 2 poles (114.2628, 145.8792) (114.2628, 146.3756) (114.1295, 147.4797) (113.9813, 147.9688) knots 0 0 0 1 2 2 2
  line L214 (113.9813, 147.9688) -> (114.8482, 147.9688)
  spline S151 degree 2 poles (114.8482, 147.9688) (114.9742, 147.4501) (115.0705, 146.3905) (115.0705, 145.8717) knots 0 0 0 1 2 2 2
  spline S152 degree 2 poles (115.0705, 145.8717) (115.0705, 143.7006) (112.0843, 140.8477) (109.7131, 140.8477) knots 0 0 0 1 2 2 2
  spline S153 degree 2 poles (109.7131, 140.8477) (107.4604, 140.8477) (104.363, 143.7895) (104.363, 145.9014) knots 0 0 0 1 2 2 2
  spline S154 degree 2 poles (104.363, 145.9014) (104.363, 148.1615) (107.2752, 150.7179) (109.6093, 150.7179) knots 0 0 0 1 2 2 2
  line L215 (111.1803, 147.0574) -> (108.0013, 147.0574)
  spline S155 degree 2 poles (108.0013, 147.0574) (107.8235, 146.7165) (107.6679, 146.1385) (107.6679, 145.8199) knots 0 0 0 1 2 2 2
  spline S156 degree 2 poles (107.6679, 145.8199) (107.6679, 145.1233) (108.7053, 144.2786) (109.7946, 144.2786) knots 0 0 0 1 2 2 2
  spline S157 degree 2 poles (109.7946, 144.2786) (110.7727, 144.2786) (111.8175, 144.9159) (111.8175, 145.6198) knots 0 0 0 1 2 2 2
  spline S158 degree 2 poles (111.8175, 145.6198) (111.8175, 145.9903) (111.4618, 146.7239) (111.1803, 147.0574) knots 0 0 0 1 2 2 2
  line L216 (113.6849, 157.6463) -> (113.6849, 156.4903)
  line L217 (113.6849, 156.4903) -> (112.929, 156.4903)
  spline S159 degree 2 poles (112.929, 156.4903) (113.3959, 155.9568) (113.8775, 155.0009) (113.8775, 154.4081) knots 0 0 0 1 2 2 2
  spline S160 degree 2 poles (113.8775, 154.4081) (113.8775, 153.9635) (113.5811, 153.1706) (113.2625, 152.8817) knots 0 0 0 1 2 2 2
  spline S161 degree 2 poles (113.2625, 152.8817) (112.9439, 152.5853) (111.9731, 152.2592) (111.2766, 152.2592) knots 0 0 0 1 2 2 2
  line L218 (111.2766, 152.2592) -> (106.8232, 152.2592)
  line L219 (106.8232, 152.2592) -> (106.8232, 153.4152)
  line L220 (106.8232, 153.4152) -> (110.7357, 153.4152)
  spline S162 degree 2 poles (110.7357, 153.4152) (111.284, 153.4152) (112.0028, 153.4967) (112.2695, 153.6375) knots 0 0 0 1 2 2 2
  spline S163 degree 2 poles (112.2695, 153.6375) (112.5363, 153.7783) (112.7808, 154.2599) (112.7808, 154.7119) knots 0 0 0 1 2 2 2
  spline S164 degree 2 poles (112.7808, 154.7119) (112.7808, 155.1343) (112.2992, 156.0902) (111.9509, 156.4903) knots 0 0 0 1 2 2 2
  line L221 (111.9509, 156.4903) -> (106.8232, 156.4903)
  line L222 (106.8232, 156.4903) -> (106.8232, 157.6463)
  line L223 (106.8232, 157.6463) -> (113.6849, 157.6463)
  spline S165 degree 2 poles (113.8405, 162.0479) (113.8405, 161.3365) (113.4033, 160.1583) (112.9587, 159.7359) knots 0 0 0 1 2 2 2
  spline S166 degree 2 poles (112.9587, 159.7359) (112.5215, 159.3136) (111.1728, 158.8467) (110.2688, 158.8467) knots 0 0 0 1 2 2 2
  spline S167 degree 2 poles (110.2688, 158.8467) (109.3648, 158.8467) (108.0458, 159.3284) (107.6012, 159.7359) knots 0 0 0 1 2 2 2
  spline S168 degree 2 poles (107.6012, 159.7359) (107.1492, 160.1435) (106.6675, 161.3513) (106.6675, 162.0479) knots 0 0 0 1 2 2 2
  spline S169 degree 2 poles (106.6675, 162.0479) (106.6675, 162.611) (106.9862, 163.6633) (107.1937, 164.0708) knots 0 0 0 1 2 2 2
  line L224 (107.1937, 164.0708) -> (108.4904, 164.0708)
  line L225 (108.4904, 164.0708) -> (108.4904, 164.0041)
  spline S170 degree 2 poles (108.4904, 164.0041) (108.3867, 163.8782) (108.1199, 163.4928) (107.9791, 163.2187) knots 0 0 0 1 2 2 2
  spline S171 degree 2 poles (107.9791, 163.2187) (107.8606, 162.9741) (107.6753, 162.3221) (107.6753, 162.0257) knots 0 0 0 1 2 2 2
  spline S172 degree 2 poles (107.6753, 162.0257) (107.6753, 161.129) (109.0313, 160.0398) (110.2688, 160.0398) knots 0 0 0 1 2 2 2
  spline S173 degree 2 poles (110.2688, 160.0398) (111.4767, 160.0398) (112.8327, 161.092) (112.8327, 162.0257) knots 0 0 0 1 2 2 2
  spline S174 degree 2 poles (112.8327, 162.0257) (112.8327, 162.5888) (112.3659, 163.6114) (112.0028, 164.0041) knots 0 0 0 1 2 2 2
  line L226 (112.0028, 164.0041) -> (112.0028, 164.0708)
  line L227 (112.0028, 164.0708) -> (113.2995, 164.0708)
  spline S175 degree 2 poles (113.2995, 164.0708) (113.381, 163.9004) (113.6108, 163.3817) (113.6626, 163.1742) knots 0 0 0 1 2 2 2
  spline S176 degree 2 poles (113.6626, 163.1742) (113.7515, 162.8778) (113.8405, 162.411) (113.8405, 162.0479) knots 0 0 0 1 2 2 2
  spline S177 degree 2 poles (113.8479, 166.9756) (113.8479, 166.2864) (113.4774, 165.0934) (113.2699, 164.7007) knots 0 0 0 1 2 2 2
  line L228 (113.2699, 164.7007) -> (111.9731, 164.7007)
  line L229 (111.9731, 164.7007) -> (111.9731, 164.76)
  spline S178 degree 2 poles (111.9731, 164.76) (112.0917, 164.9082) (112.3733, 165.3083) (112.5289, 165.6418) knots 0 0 0 1 2 2 2
  spline S179 degree 2 poles (112.5289, 165.6418) (112.6697, 165.9307) (112.8772, 166.6421) (112.8772, 167.02) knots 0 0 0 1 2 2 2
  spline S180 degree 2 poles (112.8772, 167.02) (112.8772, 167.2942) (112.7512, 167.9241) (112.6474, 168.0723) knots 0 0 0 1 2 2 2
  spline S181 degree 2 poles (112.6474, 168.0723) (112.5067, 168.2871) (112.188, 168.4798) (111.862, 168.4798) knots 0 0 0 1 2 2 2
  spline S182 degree 2 poles (111.862, 168.4798) (111.4544, 168.4798) (111.0321, 168.0352) (110.8913, 167.4646) knots 0 0 0 1 2 2 2
  spline S183 degree 2 poles (110.8913, 167.4646) (110.8394, 167.2423) (110.6912, 166.531) (110.6097, 166.2272) knots 0 0 0 1 2 2 2
  spline S184 degree 2 poles (110.6097, 166.2272) (110.38, 165.4417) (109.4315, 164.7303) (108.7572, 164.7303) knots 0 0 0 1 2 2 2
  spline S185 degree 2 poles (108.7572, 164.7303) (107.8235, 164.7303) (106.6601, 166.1308) (106.6601, 167.2868) knots 0 0 0 1 2 2 2
  spline S186 degree 2 poles (106.6601, 167.2868) (106.6601, 167.8574) (106.9417, 169.0133) (107.1566, 169.4061) knots 0 0 0 1 2 2 2
  line L230 (107.1566, 169.4061) -> (108.3941, 169.4061)
  line L231 (108.3941, 169.4061) -> (108.3941, 169.3468)
  spline S187 degree 2 poles (108.3941, 169.3468) (108.0384, 168.9022) (107.6308, 167.8203) (107.6308, 167.2646) knots 0 0 0 1 2 2 2
  spline S188 degree 2 poles (107.6308, 167.2646) (107.6308, 166.694) (108.1125, 165.9085) (108.5942, 165.9085) knots 0 0 0 1 2 2 2
  spline S189 degree 2 poles (108.5942, 165.9085) (109.0313, 165.9085) (109.4537, 166.3754) (109.5871, 166.8941) knots 0 0 0 1 2 2 2
  spline S190 degree 2 poles (109.5871, 166.8941) (109.6538, 167.146) (109.7872, 167.7833) (109.8687, 168.1315) knots 0 0 0 1 2 2 2
  spline S191 degree 2 poles (109.8687, 168.1315) (110.0613, 168.8874) (110.9431, 169.658) (111.7064, 169.658) knots 0 0 0 1 2 2 2
  spline S192 degree 2 poles (111.7064, 169.658) (112.151, 169.658) (112.9364, 169.3097) (113.2254, 168.9689) knots 0 0 0 1 2 2 2
  spline S193 degree 2 poles (113.2254, 168.9689) (113.5292, 168.6058) (113.8479, 167.6795) (113.8479, 166.9756) knots 0 0 0 1 2 2 2
  line L232 (113.6849, 176.0084) -> (113.6849, 174.8524)
  line L233 (113.6849, 174.8524) -> (112.9883, 174.8524)
  spline S194 degree 2 poles (112.9883, 174.8524) (113.2106, 174.5857) (113.507, 174.193) (113.633, 173.9262) knots 0 0 0 1 2 2 2
  spline S195 degree 2 poles (113.633, 173.9262) (113.7515, 173.6817) (113.8775, 173.1555) (113.8775, 172.8073) knots 0 0 0 1 2 2 2
  spline S196 degree 2 poles (113.8775, 172.8073) (113.8775, 172.2441) (113.4107, 171.2956) (112.9587, 170.9622) knots 0 0 0 1 2 2 2
  spline S197 degree 2 poles (112.9587, 170.9622) (112.5067, 170.6287) (111.1728, 170.2582) (110.3059, 170.2582) knots 0 0 0 1 2 2 2
  spline S198 degree 2 poles (110.3059, 170.2582) (109.4018, 170.2582) (108.0829, 170.7251) (107.5864, 171.1326) knots 0 0 0 1 2 2 2
  spline S199 degree 2 poles (107.5864, 171.1326) (107.1418, 171.5105) (106.6305, 172.5702) (106.6305, 173.1555) knots 0 0 0 1 2 2 2
  spline S200 degree 2 poles (106.6305, 173.1555) (106.6305, 173.6668) (106.8602, 174.4301) (107.0973, 174.8524) knots 0 0 0 1 2 2 2
  line L234 (107.0973, 174.8524) -> (104.1333, 174.8524)
  line L235 (104.1333, 174.8524) -> (104.1333, 176.0084)
  line L236 (104.1333, 176.0084) -> (113.6849, 176.0084)
  line L237 (112.0176, 174.8524) -> (108.0532, 174.8524)
  spline S201 degree 2 poles (108.0532, 174.8524) (107.8457, 174.4227) (107.6901, 173.7409) (107.6901, 173.3482) knots 0 0 0 1 2 2 2
  spline S202 degree 2 poles (107.6901, 173.3482) (107.6901, 172.459) (109.0239, 171.4512) (110.2836, 171.4512) knots 0 0 0 1 2 2 2
  spline S203 degree 2 poles (110.2836, 171.4512) (111.4989, 171.4512) (112.7808, 172.2219) (112.7808, 173.074) knots 0 0 0 1 2 2 2
  spline S204 degree 2 poles (112.7808, 173.074) (112.7808, 173.526) (112.3659, 174.4449) (112.0176, 174.8524) knots 0 0 0 1 2 2 2
  line L238 (113.6849, 179.4763) -> (113.6849, 178.0091)
  line L239 (113.6849, 178.0091) -> (111.9361, 178.0091)
  line L240 (111.9361, 178.0091) -> (111.9361, 179.4763)
  line L241 (111.9361, 179.4763) -> (113.6849, 179.4763)
  spline S205 degree 2 poles (113.8405, 184.4707) (113.8405, 182.8257) (111.9954, 181.0176) (110.2911, 181.0176) knots 0 0 0 1 2 2 2
  spline S206 degree 2 poles (110.2911, 181.0176) (108.6164, 181.0176) (106.6305, 182.7738) (106.6305, 184.1891) knots 0 0 0 1 2 2 2
  spline S207 degree 2 poles (106.6305, 184.1891) (106.6305, 184.8264) (107.001, 185.8119) (107.3937, 186.175) knots 0 0 0 1 2 2 2
  spline S208 degree 2 poles (107.3937, 186.175) (107.7865, 186.5455) (108.9202, 186.9382) (109.7427, 186.9382) knots 0 0 0 1 2 2 2
  line L242 (109.7427, 186.9382) -> (110.3726, 186.9382)
  line L243 (110.3726, 186.9382) -> (110.3726, 182.1884)
  spline S209 degree 2 poles (110.3726, 182.1884) (111.5656, 182.1884) (112.8327, 183.3888) (112.8327, 184.4559) knots 0 0 0 1 2 2 2
  spline S210 degree 2 poles (112.8327, 184.4559) (112.8327, 184.8338) (112.6623, 185.5674) (112.5289, 185.8638) knots 0 0 0 1 2 2 2
  spline S211 degree 2 poles (112.5289, 185.8638) (112.3807, 186.175) (112.1213, 186.6048) (112.0028, 186.7456) knots 0 0 0 1 2 2 2
  line L244 (112.0028, 186.7456) -> (112.0028, 186.8123)
  line L245 (112.0028, 186.8123) -> (113.2625, 186.8123)
  spline S212 degree 2 poles (113.2625, 186.8123) (113.344, 186.6122) (113.5811, 186.0046) (113.6478, 185.7674) knots 0 0 0 1 2 2 2
  spline S213 degree 2 poles (113.6478, 185.7674) (113.7441, 185.434) (113.8405, 184.8857) (113.8405, 184.4707) knots 0 0 0 1 2 2 2
  spline S214 degree 2 poles (109.4908, 185.8119) (109.0239, 185.7971) (108.3422, 185.6044) (108.1125, 185.4192) knots 0 0 0 1 2 2 2
  spline S215 degree 2 poles (108.1125, 185.4192) (107.8531, 185.2191) (107.579, 184.5893) (107.579, 184.1224) knots 0 0 0 1 2 2 2
  spline S216 degree 2 poles (107.579, 184.1224) (107.579, 183.663) (107.8531, 183.0183) (108.1199, 182.7516) knots 0 0 0 1 2 2 2
  spline S217 degree 2 poles (108.1199, 182.7516) (108.3941, 182.4922) (109.0536, 182.2254) (109.4908, 182.1884) knots 0 0 0 1 2 2 2
  line L246 (109.4908, 182.1884) -> (109.4908, 185.8119)
  line L247 (113.6849, 193.385) -> (113.6849, 192.229)
  line L248 (113.6849, 192.229) -> (112.9883, 192.229)
  spline S218 degree 2 poles (112.9883, 192.229) (113.2106, 191.9622) (113.507, 191.5695) (113.633, 191.3028) knots 0 0 0 1 2 2 2
  spline S219 degree 2 poles (113.633, 191.3028) (113.7515, 191.0582) (113.8775, 190.5321) (113.8775, 190.1838) knots 0 0 0 1 2 2 2
  spline S220 degree 2 poles (113.8775, 190.1838) (113.8775, 189.6207) (113.4107, 188.6722) (112.9587, 188.3387) knots 0 0 0 1 2 2 2
  spline S221 degree 2 poles (112.9587, 188.3387) (112.5067, 188.0053) (111.1728, 187.6348) (110.3059, 187.6348) knots 0 0 0 1 2 2 2
  spline S222 degree 2 poles (110.3059, 187.6348) (109.4018, 187.6348) (108.0829, 188.1016) (107.5864, 188.5092) knots 0 0 0 1 2 2 2
  spline S223 degree 2 poles (107.5864, 188.5092) (107.1418, 188.8871) (106.6305, 189.9467) (106.6305, 190.5321) knots 0 0 0 1 2 2 2
  spline S224 degree 2 poles (106.6305, 190.5321) (106.6305, 191.0434) (106.8602, 191.8066) (107.0973, 192.229) knots 0 0 0 1 2 2 2
  line L249 (107.0973, 192.229) -> (104.1333, 192.229)
  line L250 (104.1333, 192.229) -> (104.1333, 193.385)
  line L251 (104.1333, 193.385) -> (113.6849, 193.385)
  line L252 (112.0176, 192.229) -> (108.0532, 192.229)
  spline S225 degree 2 poles (108.0532, 192.229) (107.8457, 191.7992) (107.6901, 191.1175) (107.6901, 190.7248) knots 0 0 0 1 2 2 2
  spline S226 degree 2 poles (107.6901, 190.7248) (107.6901, 189.8356) (109.0239, 188.8278) (110.2836, 188.8278) knots 0 0 0 1 2 2 2
  spline S227 degree 2 poles (110.2836, 188.8278) (111.4989, 188.8278) (112.7808, 189.5984) (112.7808, 190.4506) knots 0 0 0 1 2 2 2
  spline S228 degree 2 poles (112.7808, 190.4506) (112.7808, 190.9026) (112.3659, 191.8215) (112.0176, 192.229) knots 0 0 0 1 2 2 2
  line L253 (113.6849, 200.3949) -> (113.6849, 199.2389)
  line L254 (113.6849, 199.2389) -> (112.929, 199.2389)
  spline S229 degree 2 poles (112.929, 199.2389) (113.3959, 198.7054) (113.8775, 197.7495) (113.8775, 197.1567) knots 0 0 0 1 2 2 2
  spline S230 degree 2 poles (113.8775, 197.1567) (113.8775, 196.7121) (113.5811, 195.9192) (113.2625, 195.6302) knots 0 0 0 1 2 2 2
  spline S231 degree 2 poles (113.2625, 195.6302) (112.9439, 195.3338) (111.9731, 195.0078) (111.2766, 195.0078) knots 0 0 0 1 2 2 2
  line L255 (111.2766, 195.0078) -> (106.8232, 195.0078)
  line L256 (106.8232, 195.0078) -> (106.8232, 196.1637)
  line L257 (106.8232, 196.1637) -> (110.7357, 196.1637)
  spline S232 degree 2 poles (110.7357, 196.1637) (111.284, 196.1637) (112.0028, 196.2453) (112.2695, 196.386) knots 0 0 0 1 2 2 2
  spline S233 degree 2 poles (112.2695, 196.386) (112.5363, 196.5268) (112.7808, 197.0085) (112.7808, 197.4605) knots 0 0 0 1 2 2 2
  spline S234 degree 2 poles (112.7808, 197.4605) (112.7808, 197.8829) (112.2992, 198.8388) (111.9509, 199.2389) knots 0 0 0 1 2 2 2
  line L258 (111.9509, 199.2389) -> (106.8232, 199.2389)
  line L259 (106.8232, 199.2389) -> (106.8232, 200.3949)
  line L260 (106.8232, 200.3949) -> (113.6849, 200.3949)
  line L261 (128.7402, 99.5664) -> (128.7402, 98.3511)
  line L262 (128.7402, 98.3511) -> (120.8633, 98.3511)
  line L263 (120.8633, 98.3511) -> (126.2208, 95.9651)
  line L264 (126.2208, 95.9651) -> (126.2208, 95.2241)
  line L265 (126.2208, 95.2241) -> (120.8633, 92.8603)
  line L266 (120.8633, 92.8603) -> (128.7402, 92.8603)
  line L267 (128.7402, 92.8603) -> (128.7402, 91.7265)
  line L268 (128.7402, 91.7265) -> (119.5962, 91.7265)
  line L269 (119.5962, 91.7265) -> (119.5962, 93.3864)
  line L270 (119.5962, 93.3864) -> (124.6869, 95.6687)
  line L271 (124.6869, 95.6687) -> (119.5962, 97.8769)
  line L272 (119.5962, 97.8769) -> (119.5962, 99.5664)
  line L273 (119.5962, 99.5664) -> (128.7402, 99.5664)
  spline S235 degree 2 poles (128.9329, 104.6126) (128.9329, 103.8049) (128.5105, 102.6045) (128.0881, 102.1821) knots 0 0 0 1 2 2 2
  spline S236 degree 2 poles (128.0881, 102.1821) (127.6139, 101.7004) (126.2801, 101.3077) (125.3019, 101.3077) knots 0 0 0 1 2 2 2
  line L274 (125.3019, 101.3077) -> (119.5962, 101.3077)
  line L275 (119.5962, 101.3077) -> (119.5962, 102.523)
  line L276 (119.5962, 102.523) -> (125.3019, 102.523)
  spline S237 degree 2 poles (125.3019, 102.523) (125.9392, 102.523) (126.7988, 102.686) (127.1471, 102.9157) knots 0 0 0 1 2 2 2
  spline S238 degree 2 poles (127.1471, 102.9157) (127.5176, 103.1602) (127.8955, 104.005) (127.8955, 104.6126) knots 0 0 0 1 2 2 2
  spline S239 degree 2 poles (127.8955, 104.6126) (127.8955, 105.1832) (127.5176, 106.0724) (127.1471, 106.3169) knots 0 0 0 1 2 2 2
  spline S240 degree 2 poles (127.1471, 106.3169) (126.7988, 106.5466) (125.9466, 106.7096) (125.3316, 106.7096) knots 0 0 0 1 2 2 2
  line L277 (125.3316, 106.7096) -> (119.5962, 106.7096)
  line L278 (119.5962, 106.7096) -> (119.5962, 107.9249)
  line L279 (119.5962, 107.9249) -> (125.3019, 107.9249)
  spline S241 degree 2 poles (125.3019, 107.9249) (126.2578, 107.9249) (127.6213, 107.5396) (128.0881, 107.0505) knots 0 0 0 1 2 2 2
  spline S242 degree 2 poles (128.0881, 107.0505) (128.5179, 106.6133) (128.9329, 105.4573) (128.9329, 104.6126) knots 0 0 0 1 2 2 2
  spline S243 degree 2 poles (128.9032, 112.2153) (128.9032, 111.2224) (128.4883, 109.8293) (128.1919, 109.2142) knots 0 0 0 1 2 2 2
  line L280 (128.1919, 109.2142) -> (126.6654, 109.2142)
  line L281 (126.6654, 109.2142) -> (126.6654, 109.3032)
  spline S244 degree 2 poles (126.6654, 109.3032) (127.2286, 109.9034) (127.851, 111.4224) (127.851, 112.1264) knots 0 0 0 1 2 2 2
  spline S245 degree 2 poles (127.851, 112.1264) (127.851, 113.1342) (127.0137, 114.1641) (126.3245, 114.1641) knots 0 0 0 1 2 2 2
  spline S246 degree 2 poles (126.3245, 114.1641) (125.7762, 114.1641) (125.0945, 113.6232) (124.924, 113.0378) knots 0 0 0 1 2 2 2
  spline S247 degree 2 poles (124.924, 113.0378) (124.8055, 112.6154) (124.6425, 111.9115) (124.5091, 111.3854) knots 0 0 0 1 2 2 2
  spline S248 degree 2 poles (124.5091, 111.3854) (124.3831, 110.9111) (124.0052, 110.1627) (123.7014, 109.8737) knots 0 0 0 1 2 2 2
  spline S249 degree 2 poles (123.7014, 109.8737) (123.3976, 109.5921) (122.5825, 109.2809) (122.0489, 109.2809) knots 0 0 0 1 2 2 2
  spline S250 degree 2 poles (122.0489, 109.2809) (120.9374, 109.2809) (119.4332, 111.0149) (119.4332, 112.3561) knots 0 0 0 1 2 2 2
  spline S251 degree 2 poles (119.4332, 112.3561) (119.4332, 113.1267) (119.737, 114.4902) (120.026, 115.0756) knots 0 0 0 1 2 2 2
  line L282 (120.026, 115.0756) -> (121.4784, 115.0756)
  line L283 (121.4784, 115.0756) -> (121.4784, 114.9867)
  spline S252 degree 2 poles (121.4784, 114.9867) (121.0782, 114.5495) (120.4854, 113.186) (120.4854, 112.4376) knots 0 0 0 1 2 2 2
  spline S253 degree 2 poles (120.4854, 112.4376) (120.4854, 111.5929) (121.2783, 110.548) (121.923, 110.548) knots 0 0 0 1 2 2 2
  spline S254 degree 2 poles (121.923, 110.548) (122.5009, 110.548) (123.1901, 111.1631) (123.3457, 111.7411) knots 0 0 0 1 2 2 2
  spline S255 degree 2 poles (123.3457, 111.7411) (123.4494, 112.1264) (123.7162, 113.2453) (123.8273, 113.6158) knots 0 0 0 1 2 2 2
  spline S256 degree 2 poles (123.8273, 113.6158) (124.1163, 114.5569) (125.2797, 115.4313) (126.1319, 115.4313) knots 0 0 0 1 2 2 2
  spline S257 degree 2 poles (126.1319, 115.4313) (126.6728, 115.4313) (127.7102, 114.9941) (128.0733, 114.6013) knots 0 0 0 1 2 2 2
  spline S258 degree 2 poles (128.0733, 114.6013) (128.4734, 114.1641) (128.9032, 113.0526) (128.9032, 112.2153) knots 0 0 0 1 2 2 2
  line L284 (128.7402, 125.5163) -> (128.7402, 121.0555)
  line L285 (128.7402, 121.0555) -> (127.8065, 121.0555)
  line L286 (127.8065, 121.0555) -> (127.8065, 122.7153)
  line L287 (127.8065, 122.7153) -> (121.6784, 122.7153)
  line L288 (121.6784, 122.7153) -> (121.6784, 121.0555)
  line L289 (121.6784, 121.0555) -> (120.8411, 121.0555)
  spline S259 degree 2 poles (120.8411, 121.0555) (120.8411, 121.9966) (120.3076, 122.8858) (119.5666, 122.9451) knots 0 0 0 1 2 2 2